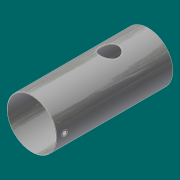
# Autodesk Inventor part: A1-19027-400-01 36in pipe
Saved by Autodesk Inventor 2017.3 (Build 213257000, 257)
## iProperties
Created: 2019-08-16
Part Number: A1-19027-400-01 36in pipe
Material: Steel, Mild
Document SubType Name: Modeling
Designer: GVD
Density: 7.85 g/cm^3
Appearance: Steel
Description: 36" STD x 84 7/16" PIPE, (GRADE TBD)
Mass: 441718 g
Surface Area: 119046 cm^2
Volume: 56269.8 cm^3
Author: GVD
Autodesk Inventor part; units mm, degrees
ref_plane "XY Plane" through (0, 0, 0) normal (0, 0, 1) x (1, 0, 0)
sketch "Sketch1" plane through (0, 0, 0) normal (0, 0, 1) x (1, 0, 0)
  circle A0 centre (0, 0) radius 457.2
  circle A1 centre (0, 0) radius 447.675
  dimension "d0" = 914.4
  dimension "d1" = 895.35
  constraints: 2 centre point, 2 coincident
  measures "d0" diameter of A0
  measures "d1" diameter of A1
extrude "Extrusion1" add sketch "Sketch1" along normal blind 2150.8313
ref_plane "Work Plane1" through (457.2, 0, 0) normal (1, 0, 0) x (0, 1, 0)
ref_plane "Work Plane2" through (0, 457.2, 0) normal (0, 1, 0) x (-1, 0, 0)
sketch "Sketch4" plane through (0, 457.2, 0) normal (0, 1, 0) x (-1, 0, 0)
  line L0 (457.2, 2150.8313) -> (-457.2, 2150.8313) construction
  circle A0 centre (0, 1916.4125) radius 66.675
  circle A1 centre (0, 724.4125) radius 165.1
  circle A2 centre (0, 724.4125) radius 177.8
  point P0 (0, 0)
  dimension "d14" = 234.4187
  dimension "d15" = 133.35
  dimension "d16" = 330.2
  dimension "d17" = 355.6
  dimension "d18" = 1192
  constraints: 3 centre point, 2 coincident, 2 vertical alignment
  measures "d14" distance from line of L0 point (0, 1916.413)
  measures "d15" diameter of A0
  measures "d16" diameter of A1
  measures "d17" diameter of A2
  measures "d18" distance of A1.centre point (0, 1916.413)
extrude "Extrusion3" cut sketch "Sketch4" against normal up to surface (457.2 mm away) contours A1
extrude_surface "ExtrusionSrf1" [suppressed]
surface extrude "ExtrusionSrf2" sketch "Sketch4" against normal up to surface (457.2 mm away) shown no curves A2
hole "Hole1" [suppressed]
pattern_circular "Circular Pattern1" count 2 over 360 about axis through (0, 0, -10) along (0, 0, 1) of "Extrusion3", "ExtrusionSrf2"
split_face "Split1"
split_face "Split2"
split "Split3" [suppressed]
split "Split4" [suppressed]
chamfer "Chamfer1" distance 7.9375 angle 37.5 1 edges at (-457.2, 0, 0) measured on face at (-456.7, 0, 0)
sketch "Sketch5" plane through (0, 457.2, 0) normal (0, 1, 0) x (-1, 0, 0)
  point P0 (0, 0)
  point P1 (0, 150.8125)
  dimension "d38" = 150.8125
  constraints: 1 vertical alignment
  measures "d38" distance of point (0, 0) point (0, 150.812)
hole "Hole2" at (0, 457.2, 150.8125) direction (0, -1, 0) diameter 17.4752 depth 22.6314 tip angle 118 taper from width 18.3226 to width 17.4752 over 13.5636 thread size "1/2" designation "1/2 - 14 NPT" standard "NPT"
pattern_circular "Circular Pattern2" count 3 over 270 about axis through (0, 0, -10) along (0, 0, 1) of "Hole2" both ways yes
ref_plane "Work Plane3" through (457.2, 0, 0) normal (1, 0, 0) x (0, 1, 0)
sketch "Sketch6" plane through (457.2, 0, 0) normal (1, 0, 0) x (0, 1, 0)
  line L0 (457.2, 2150.8313) -> (-457.2, 2150.8313) construction
  circle A0 centre (0, 2000.8125) radius 52.3875
  point P0 (0, 0)
  dimension "d51" = 104.775
  dimension "d52" = 150.0188
  constraints: 1 centre point, 1 coincident, 1 vertical alignment
  measures "d51" diameter of A0
  measures "d52" distance from line of point (0, 2000.812) L0
hole "Hole3" at (457.2, 0, 2000.8125) direction (-1, 0, 0) diameter 65.0875 depth 22.6314 tip angle 118
surface extrude "ExtrusionSrf5" sketch "Sketch6" against normal blind 25.4 shown no curves A0
split_face "Split5"
chamfer "Chamfer2" distance 7.9375 angle 37.5 1 edges at (-457.2, 0, 2150.8313) measured on face at (-456.7, 0, 2150.8312)
body "Solid1"
body "Srf1"
body "Srf2"
body "Srf3"
body "Srf4"
body "Srf5"
